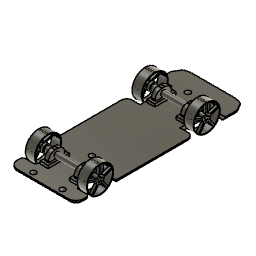
CAR BAse v6 (Autodesk Fusion 360 design; units mm, degrees)
Autodesk Fusion 360 part; units mm, degrees
note: some values were not read from the file. Set by a fixed rule: which face or edge a step refers to.
sketch "Sketch1" plane through (0, 0, 0) normal (0, 0, 1) x (1, 0, 0)
  line L0 (-50, 58.039) -> (-50, 31)
  line L1 (-50, 19) -> (-50, 18)
  line L2 (-47, 15) -> (-28, 15)
  line L3 (-25, 18) -> (-25, 19)
  line L4 (-25, 31) -> (-25, 58)
  line L5 (-25, 70) -> (-25, 70)
  line L6 (-30, 75) -> (-45, 75)
  line L7 (-50, 70) -> (-50, 70)
  arc A0 (-45, 75) -> (-50, 70) centre (-45, 70) ccw
  arc A1 (-25, 70) -> (-30, 75) centre (-30, 70) ccw
  arc A2 (-28, 15) -> (-25, 18) centre (-28, 18) ccw
  arc A3 (-50, 18) -> (-47, 15) centre (-47, 18) ccw
  line L8 (-49, 20) -> (-46, 20)
  line L9 (-45, 21) -> (-45, 29)
  line L10 (-46, 30) -> (-49, 30)
  line L11 (-26, 20) -> (-29, 20)
  line L12 (-30, 21) -> (-30, 30)
  line L13 (-30, 30) -> (-26, 30)
  line L14 (-25, 70) -> (-30, 70)
  line L15 (-30, 70) -> (-30, 60)
  line L16 (-30, 60) -> (-27, 60)
  line L17 (-48, 60.039) -> (-45, 60.039)
  line L18 (-45, 60.039) -> (-45, 70)
  line L19 (-45, 70) -> (-50, 70)
  line L20 (-44, 55) -> (-31, 55)
  line L21 (-31, 55) -> (-31, 35)
  line L22 (-31, 35) -> (-44, 35)
  line L23 (-44, 35) -> (-44, 55)
  circle A4 centre (-43, 28) radius 1
  circle A5 centre (-43, 22) radius 1
  circle A6 centre (-32, 22) radius 1
  circle A7 centre (-32, 28) radius 1
  circle A8 centre (-43, 68) radius 1
  circle A9 centre (-43, 62) radius 1
  circle A10 centre (-32, 62) radius 1
  circle A11 centre (-32, 68) radius 1
  circle A12 centre (-40, 72) radius 1
  circle A13 centre (-35, 72) radius 1
  circle A14 centre (-37.4904, 33.4419) radius 1
  circle A15 centre (-43, 17) radius 1
  circle A16 centre (-32, 17) radius 1
  arc A17 (-48, 60.039) -> (-50, 58.039) centre (-48, 58.039) ccw
  arc A18 (-25, 58) -> (-27, 60) centre (-27, 58) ccw
  arc A19 (-25, 19) -> (-26, 20) centre (-26, 19) ccw
  arc A20 (-26, 30) -> (-25, 31) centre (-26, 31) ccw
  arc A21 (-50, 31) -> (-49, 30) centre (-49, 31) ccw
  arc A22 (-49, 20) -> (-50, 19) centre (-49, 19) ccw
  arc A23 (-46, 20) -> (-45, 21) centre (-46, 21) ccw
  arc A24 (-45, 29) -> (-46, 30) centre (-46, 29) ccw
  arc A25 (-30, 21) -> (-29, 20) centre (-29, 21) ccw
  dimension "d1" = 5
  dimension "d2" = 5
  dimension "d3" = 3
  dimension "d4" = 3
  dimension "d5" = 2
  dimension "d6" = 2
  dimension "d7" = 2
  dimension "d8" = 1
  dimension "d9" = 1
  constraint vertical L0
  constraint parallel L0 L1
  constraint perpendicular L1 L2
  constraint perpendicular L2 L3
  constraint perpendicular L2 L4
  constraint tangent L6 A0
  constraint tangent L6 A1
  constraint tangent L2 A2
  constraint tangent L3 A2
  constraint tangent L1 A3
  constraint tangent L2 A3
  constraint horizontal L8
  constraint vertical L9
  constraint horizontal L10
  constraint horizontal L11
  constraint vertical L12
  constraint horizontal L13
  constraint horizontal L14
  constraint vertical L15
  constraint horizontal L16
  constraint horizontal L17
  constraint vertical L18
  constraint horizontal L19
  constraint coincident A0.centre L18.end
  constraint horizontal L20
  constraint vertical L21
  constraint horizontal L22
  constraint vertical L23
  constraint tangent L17 A17
  constraint tangent L0 A17
  constraint tangent L16 A18
  constraint tangent L4 A18
  constraint tangent L3 A19
  constraint tangent L11 A19
  constraint tangent L13 A20
  constraint tangent L4 A20
  constraint tangent L10 A21
  constraint tangent L0 A21
  constraint equal A20 A21
  constraint tangent L1 A22
  constraint tangent L8 A22
  constraint equal A20 A22
  constraint tangent L8 A23
  constraint tangent L9 A23
  constraint equal A20 A23
  constraint tangent L9 A24
  constraint tangent L10 A24
  constraint equal A20 A24
  constraint tangent L11 A25
  constraint tangent L12 A25
  constraint equal A20 A25
  measures "d1" radius of A0
  measures "d2" radius of A1
  measures "d3" radius of A2
  measures "d4" radius of A3
  measures "d5" diameter of A14
  measures "d6" radius of A17
  measures "d7" radius of A18
  measures "d8" radius of A19
  measures "d9" radius of A20
extrude "Extrude1" add sketch "Sketch1" along normal blind 1.5 makes body 1
sketch "Sketch2" plane through (0, 0, 0) normal (0, 0, 1) x (1, 0, 0)
  circle A0 centre (0, 0) radius 1
  line L0 (0, 0) -> (0, 5)
  circle A1 centre (0, 5) radius 1
  dimension "d12" = 2
  dimension "d13" = 5
  dimension "d14" = 2
  constraint coincident A0.centre L0.start
  constraint vertical L0
  constraint coincident L0.end A1.centre
  measures "d12" diameter of A0
  measures "d13" distance of A0.centre L0.end
  measures "d14" diameter of A1
extrude "Extrude2" add sketch "Sketch2" along normal blind 1.5 separate body makes body 2 at (0.995, 5.0996, 1) makes body 3 at (0.995, -0.0996, 0.5)
sketch "Sketch3" plane through (0, 0, 1.5) normal (0, 0, 1) x (-1, 0, 0)
  circle A0 centre (0, 0) radius 1
  line L0 (-1.5, -6.5) -> (1.5, -6.5)
  line L1 (1.5, -6.5) -> (1.5, 1.5)
  line L2 (1.5, 1.5) -> (-1.5, 1.5)
  line L3 (-1.5, 1.5) -> (-1.5, -6.5)
  dimension "d20" = 3
  dimension "d21" = 8
  constraint perpendicular L0 L1
  constraint perpendicular L1 L2
  constraint perpendicular L0 L3
  measures "d20" distance of L0.start L0.end
  measures "d21" distance of L0.end L1.end
extrude "Extrude3" add sketch "Sketch3" along normal blind 1 contours A0 | L0 L1 L2 L3 bodies 2 3
sketch "Sketch4" plane through (0, 0, 2.5) normal (0, 0, 1) x (-1, 0, 0)
  line L0 (-1.5, 1.5) -> (-1.5, -6.5)
  line L1 (-1.5, -6.5) -> (1.5, -6.5)
  line L2 (1.5, -6.5) -> (1.5, 1.5)
  line L3 (1.5, 1.5) -> (-1.5, 1.5)
  line L4 (0.75, -4.5) -> (0.75, -0.5)
  line L5 (-0.75, -0.5) -> (-0.75, -4.5)
  line L6 (-0.75, -4.5) -> (-0.75, -5.5)
  line L7 (-0.75, -5.5) -> (0.75, -5.5)
  line L8 (0.75, -5.5) -> (0.75, -4.5)
  line L9 (0.75, -0.5) -> (0.75, 0.5)
  line L10 (0.75, 0.5) -> (0, 0.5)
  line L11 (-0.75, -0.5) -> (-0.75, 0.5)
  line L12 (-0.75, 0.5) -> (0, 0.5)
  dimension "d24" = 1
  dimension "d25" = 1.5
  dimension "d26" = 1
  constraint perpendicular L6 L7
  measures "d24" distance of L5.end L6.end
  measures "d25" distance of L6.end L7.end
  measures "d26" distance of L4.end L9.end
extrude "Extrude4" add sketch "Sketch4" along normal blind 3 contours L4 L5 L6 L7 L8 L9 L10 L11 L12 bodies 2
fillet "Fillet1" radius 2.5 2 edges at (0, 5.5, 5.5) (0, -0.5, 5.5) on bodies 2
hole "Hole1" at (-0.75, 2.502, 3.6803) direction (1, 0, 0) diameter 2 depth 2 tip angle 118 bodies 2
copy_body "Body->Comp1" bodies 2 removing the originals makes body 4 in component "tengely tartó"
move_face "MoveFace1" to x (1, 0, 0) y (0, 1, 0) z (0, 0, 1) at (0, 0.5, 0) 1 faces at (0.995, 5.0996, 1) on bodies 4 in component "tengely tartó"
move_face "MoveFace2" to x (1, 0, 0) y (0, 1, 0) z (0, 0, 1) at (0, -0.5, 0) 1 faces at (0.995, -0.0996, 0.5) on bodies 4 in component "tengely tartó"
copy_body "Body->Comp2" bodies 1 removing the originals makes body 5 in component "alap"
move_body "Move1" bodies 5 to x (1, 0, 0) y (0, 1, 0) z (0, 0, 1) at (0, 0, 4) in component "alap"
move_body "Move1'" bodies 4 to x (1, 0, 0) y (0, 1, 0) z (0, 0, 1) at (-21, 25.94, 0) in component "tengely tartó"
move_face "OffsetFaces1" offset 20 1 faces at (-39.6667, 55, 4.5) on bodies 5 in component "alap"
cylinder "CylinderPrimitive1" add diameter 2 height -17 placed x (0, 0, -1) y (0, 1, 0) z (1, 0, 0) at (0, -76.2033, 52.8252) separate body makes body 6
move_face "MoveFace1'" to x (1, 0, 0) y (0, 1, 0) z (0, 0, 1) at (-2, 0, 0) 1 faces at (-11.3333, -76.0051, 53.8054) on bodies 6
move_body "Move1''" bodies 6 to x (1, 0, 0) y (0, 1, 0) z (0, 0, 1) at (-29, 101, -49)
move_body "Move2" bodies 6 to x (1, 0, 0) y (0, 1, 0) z (0, 0, 1) at (0, 0, 8)
copy_body "Body->Comp3" bodies 6 removing the originals makes body 7 in component "tengely"
move_face "MoveFace1''" to x (1, 0, 0) y (0, 1, 0) z (0, 0, 1) at (0, 0, -8) 1 faces at (-34.6667, 24.6972, 10.8302) on bodies 7 in component "tengely"
sketch "Sketch6" plane through (-29, 0, 0) normal (1, 0, 0) x (0, 1, 0)
  circle A0 centre (65.0267, 3.6652) radius 1
sketch "Sketch7" plane through (0, 0, 0) normal (0, 0, 1) x (1, 0, 0)
  circle A0 centre (0, 0) radius 5
  line L0 (0, 0) -> (5, 0) construction
  line L1 (0, 0) -> (-5, 0) construction
  line L2 (-2.4394, 0.5823) -> (-4.5237, 1.4488)
  line L3 (-4.5113, 1.4868) -> (-2.3158, 0.9628)
  line L4 (-2.4394, 0.5823) -> (-1.459, 0.3483)
  line L5 (-1.3851, 0.5758) -> (-2.3158, 0.9628)
  line L6 (-1.6313, -1.905) -> (-2.8081, -3.831)
  line L7 (-2.7758, -3.8546) -> (-1.3077, -2.1401)
  line L8 (-1.3077, -2.1401) -> (-0.7821, -1.28)
  line L9 (-0.9756, -1.1394) -> (-1.6313, -1.905)
  line L10 (1.3077, -2.1401) -> (2.7758, -3.8546)
  line L11 (2.8081, -3.831) -> (1.6313, -1.905)
  line L12 (1.3077, -2.1401) -> (0.7821, -1.28)
  line L13 (0.9756, -1.1394) -> (1.6313, -1.905)
  line L14 (-0.2, 2.5) -> (-0.1196, 1.4952)
  line L15 (0.1196, 1.4952) -> (0.2, 2.5)
  line L16 (0.2, 2.5) -> (0.02, 4.75)
  line L17 (-0.02, 4.75) -> (-0.2, 2.5)
  line L18 (2.3158, 0.9628) -> (1.3851, 0.5758)
  line L19 (1.459, 0.3483) -> (2.4394, 0.5823)
  line L20 (2.4394, 0.5823) -> (4.5237, 1.4488)
  line L21 (4.5113, 1.4868) -> (2.3158, 0.9628)
  line L22 (0.5701, 0.1853) -> (0, 0)
  circle A1 centre (-0.7133, -0.2318) radius 0.25
  circle A2 centre (0, -0.75) radius 0.25
  circle A3 centre (0.7133, -0.2318) radius 0.25
  circle A4 centre (0.4566, 0.595) radius 0.25
  circle A5 centre (-0.4408, 0.6068) radius 0.25
  arc A6 (-0.7821, -1.28) -> (0.7821, -1.28) centre (0, 0) ccw
  arc A7 (0.9756, -1.1394) -> (1.459, 0.3483) centre (0, 0) ccw
  arc A8 (1.3851, 0.5758) -> (0.1196, 1.4952) centre (0, 0) ccw
  arc A9 (-0.1196, 1.4952) -> (-1.3851, 0.5758) centre (0, 0) ccw
  arc A10 (-1.459, 0.3483) -> (-0.9756, -1.1394) centre (0, 0) ccw
  arc A11 (-0.02, 4.75) -> (-4.5113, 1.4868) centre (0, 0) ccw
  arc A12 (4.5113, 1.4868) -> (0.02, 4.75) centre (0, 0) ccw
  arc A13 (2.8081, -3.831) -> (4.5237, 1.4488) centre (0, 0) ccw
  arc A14 (-4.5237, 1.4488) -> (-2.8081, -3.831) centre (0, 0) ccw
  arc A15 (-2.7758, -3.8546) -> (2.7758, -3.8546) centre (0, 0) ccw
  dimension "d50" = 10
  dimension "d54" = 3
  dimension "d61" = 9.5
  dimension "d73" = 0.75
  dimension "d74" = 0.5
  dimension "d75" = 0.5
  dimension "d76" = 0.5
  dimension "d77" = 0.5
  dimension "d78" = 0.5
  constraint coincident A0.centre L0.start
  constraint concentric A0 A6
  constraint horizontal L0
  constraint horizontal L1
  constraint concentric A6 A14
  constraint coincident L17.start A14
  constraint coincident L21.start A14
  constraint coincident L11.start A14
  constraint coincident L7.start A14
  constraint coincident L4.end A6
  constraint coincident L5.start A6
  constraint coincident L15.start A6
  constraint coincident L14.end A6
  constraint coincident L18.end A6
  constraint coincident L19.start A6
  constraint coincident L13.start A6
  constraint concentric A6 A7
  constraint concentric A7 A8
  constraint concentric A8 A9
  constraint concentric A9 A10
  constraint concentric A11 A14
  constraint concentric A12 A14
  constraint concentric A13 A14
  constraint concentric A14 A15
  measures "d50" diameter of A0
  measures "d54" diameter of A6
  measures "d61" diameter of A14
  measures "d73" distance of A0.centre A1.centre
  measures "d74" diameter of A1
  measures "d75" diameter of A2
  measures "d76" diameter of A3
  measures "d77" diameter of A4
  measures "d78" diameter of A5
sketch "Sketch8" plane through (0, 0, 0.5) normal (0, 0, 1) x (-1, 0, 0)
  circle A0 centre (0.7133, 0.2318) radius 0.25
  line L0 (2.7758, 3.8546) -> (1.3077, 2.1401)
  line L1 (1.3077, 2.1401) -> (0.7821, 1.28)
  arc A1 (0.7821, 1.28) -> (-0.7821, 1.28) centre (0, 0) ccw
  line L2 (-0.7821, 1.28) -> (-1.3077, 2.1401)
  line L3 (-1.3077, 2.1401) -> (-2.7758, 3.8546)
  arc A2 (2.7758, 3.8546) -> (-2.7758, 3.8546) centre (0, 0) ccw
  line L4 (4.5237, -1.4488) -> (2.4394, -0.5823)
  line L5 (2.4394, -0.5823) -> (1.459, -0.3483)
  arc A3 (1.459, -0.3483) -> (0.9756, 1.1394) centre (0, 0) ccw
  line L6 (0.9756, 1.1394) -> (1.6313, 1.905)
  line L7 (1.6313, 1.905) -> (2.8081, 3.831)
  arc A4 (4.5237, -1.4488) -> (2.8081, 3.831) centre (0, 0) ccw
  line L8 (-1.6313, 1.905) -> (-0.9756, 1.1394)
  arc A5 (-0.9756, 1.1394) -> (-1.459, -0.3483) centre (0, 0) ccw
  line L9 (-1.459, -0.3483) -> (-2.4394, -0.5823)
  line L10 (-2.4394, -0.5823) -> (-4.5237, -1.4488)
  arc A6 (-2.8081, 3.831) -> (-4.5237, -1.4488) centre (0, 0) ccw
  line L11 (-2.8081, 3.831) -> (-1.6313, 1.905)
  line L12 (-4.5113, -1.4868) -> (-2.3158, -0.9628)
  line L13 (-2.3158, -0.9628) -> (-1.3851, -0.5758)
  arc A7 (-1.3851, -0.5758) -> (-0.1196, -1.4952) centre (0, 0) ccw
  line L14 (-0.1196, -1.4952) -> (-0.2, -2.5)
  line L15 (-0.2, -2.5) -> (-0.02, -4.75)
  arc A8 (-4.5113, -1.4868) -> (-0.02, -4.75) centre (0, 0) ccw
  line L16 (0.02, -4.75) -> (0.2, -2.5)
  line L17 (0.2, -2.5) -> (0.1196, -1.4952)
  arc A9 (0.1196, -1.4952) -> (1.3851, -0.5758) centre (0, 0) ccw
  line L18 (1.3851, -0.5758) -> (2.3158, -0.9628)
  line L19 (2.3158, -0.9628) -> (4.5113, -1.4868)
  arc A10 (0.02, -4.75) -> (4.5113, -1.4868) centre (0, 0) ccw
  circle A11 centre (0.4408, -0.6068) radius 0.25
  circle A12 centre (-0.4566, -0.595) radius 0.25
  circle A13 centre (-0.7133, 0.2318) radius 0.25
  circle A14 centre (0, 0.75) radius 0.25
  circle A15 centre (0, 0) radius 5
  line L20 (2.8081, 3.831) -> (2.7758, 3.8546)
  line L21 (-2.7758, 3.8546) -> (-2.8081, 3.831)
  line L22 (-4.5113, -1.4868) -> (-4.5237, -1.4488)
  line L23 (0.02, -4.75) -> (-0.02, -4.75)
  line L24 (4.5113, -1.4868) -> (4.5237, -1.4488)
  line L25 (1.459, -0.3483) -> (1.3851, -0.5758)
  line L26 (0.1196, -1.4952) -> (-0.1196, -1.4952)
  line L27 (-1.3851, -0.5758) -> (-1.459, -0.3483)
  line L28 (-0.9756, 1.1394) -> (-0.7821, 1.28)
  line L29 (0.7821, 1.28) -> (0.9756, 1.1394)
  constraint coincident L7.end A4.end
  constraint coincident L0.start A2.start
  constraint coincident L3.end A2.end
  constraint coincident A6.start L11.start
  constraint coincident L12.start A8.start
  constraint coincident L10.end A6.end
  constraint coincident L16.start A10.start
  constraint coincident L15.end A8.end
  constraint horizontal L23
  constraint coincident L19.end A10.end
  constraint coincident L4.start A4.start
  constraint coincident L5.end A3.start
  constraint coincident A9.end L18.start
  constraint coincident L17.end A9.start
  constraint coincident A7.end L14.start
  constraint coincident L13.end A7.start
  constraint coincident A5.end L9.start
  constraint coincident L8.end A5.start
  constraint coincident A1.end L2.start
  constraint coincident L1.end A1.start
  constraint coincident A3.end L6.start
sketch "Sketch9" plane through (0, 0, 1.8) normal (0, 0, 1) x (-1, 0, 0)
  arc A0 (0.02, -4.75) -> (4.5113, -1.4868) centre (0, 0) ccw
  line L0 (0.02, -4.75) -> (-0.02, -4.75)
  arc A1 (-4.5113, -1.4868) -> (-0.02, -4.75) centre (0, 0) ccw
  line L1 (-4.5113, -1.4868) -> (-4.5237, -1.4488)
  arc A2 (-2.8081, 3.831) -> (-4.5237, -1.4488) centre (0, 0) ccw
  line L2 (-2.8081, 3.831) -> (-2.7758, 3.8546)
  arc A3 (2.7758, 3.8546) -> (-2.7758, 3.8546) centre (0, 0) ccw
  line L3 (2.7758, 3.8546) -> (2.8081, 3.831)
  arc A4 (4.5237, -1.4488) -> (2.8081, 3.831) centre (0, 0) ccw
  line L4 (4.5237, -1.4488) -> (4.5113, -1.4868)
  circle A5 centre (0, 0) radius 5
sketch "Sketch10" plane through (-29, 0, 0) normal (1, 0, 0) x (0, 1, 0)
  circle A0 centre (25.0267, 3.6652) radius 1
  circle A1 centre (25.0267, 3.6652) radius 1.5
  line L0 (26.0267, 3.6652) -> (26.5267, 3.6652) construction
  dimension "d85" = 3
  constraint concentric A0 A1
  constraint horizontal L0
  constraint coincident A0 L0.start
  measures "d85" diameter of A1
extrude "Extrude1'" add sketch "Sketch10" along normal blind 1 contours A0 | A1 sketch seen with x (1, 0, 0) y (0, 1, 0) z (0, 0, 1) at (0, -0.23, 0.16) bodies 7 in component "tengely"
sketch "Sketch11" plane through (-28, 0, 0) normal (1, 0, 0) x (0, 1, 0)
  circle A0 centre (25.0267, 3.6652) radius 1.5
sketch "Sketch12" plane through (-46, 0, 0) normal (-1, 0, 0) x (0, -1, 0)
  circle A0 centre (-25.0267, 3.6652) radius 1
  circle A1 centre (-25.0267, 3.6652) radius 1.5
  dimension "d95" = 3
  constraint concentric A0 A1
  measures "d95" diameter of A1
extrude "Extrude2'" add sketch "Sketch12" along normal blind 1 contours A0 | A1 sketch seen with x (1, 0, 0) y (0, 1, 0) z (0, 0, 1) at (0, -0.23, 0.16) bodies 7 in component "tengely"
sketch "Sketch13" plane through (-28, 0, 0) normal (1, 0, 0) x (0, 1, 0)
  circle A0 centre (65.0267, 3.6652) radius 1.5
  line L0 (65.0267, 3.6652) -> (66.5267, 3.6652) construction
  line L1 (65.0267, 3.6652) -> (66.5267, 3.6652) construction
  line L2 (65.0267, 3.6652) -> (66.5267, 3.6652) construction
  line L3 (65.0267, 3.6652) -> (65.0267, 4.4152)
  line L4 (65.0267, 3.6652) -> (65.74, 3.897)
  line L5 (65.0267, 3.6652) -> (65.4673, 3.0583)
  line L6 (65.0267, 3.6652) -> (64.5862, 3.0583)
  line L7 (65.0267, 3.6652) -> (64.3135, 3.8974)
  circle A1 centre (64.5862, 3.0583) radius 0.25
  circle A2 centre (65.4673, 3.0583) radius 0.25
  circle A3 centre (65.0267, 4.4152) radius 0.25
  circle A4 centre (65.74, 3.897) radius 0.25
  circle A5 centre (64.3135, 3.8974) radius 0.25
  dimension "d107" = 0.5
  dimension "d108" = 0.5
  dimension "d110" = 0.5
  dimension "d111" = 0.5
  dimension "d112" = 0.5
  constraint coincident A0.centre L0.start
  constraint horizontal L0
  constraint horizontal L1
  constraint horizontal L2
  constraint coincident L6.end A1.centre
  constraint coincident L5.end A2.centre
  constraint coincident L3.end A3.centre
  constraint coincident L4.end A4.centre
  constraint coincident L7.end A5.centre
  measures "d107" diameter of A1
  measures "d108" diameter of A2
  measures "d110" diameter of A3
  measures "d111" diameter of A4
  measures "d112" diameter of A5
extrude "Extrude3'" add sketch "Sketch13" along normal blind 1.5 contours A1 | A2 | A3 | A4 | A5 sketch seen with x (1, 0, 0) y (0, 1, 0) z (0, 0, 1) at (0, -40.23, 0.16) bodies 7 in component "tengely"
sketch "Sketch14" plane through (-47, 0, 0) normal (-1, 0, 0) x (0, -1, 0)
  circle A0 centre (-65.0267, 3.6652) radius 1.5
  line L0 (-65.0267, 3.6652) -> (-65.0267, 4.4152)
  line L1 (-65.0267, 3.6652) -> (-65.74, 3.8969)
  line L2 (-65.0267, 3.6652) -> (-65.468, 3.0588)
  line L3 (-65.0267, 3.6652) -> (-64.5854, 3.0588)
  line L4 (-65.0267, 3.6652) -> (-64.3134, 3.8969)
  circle A1 centre (-65.468, 3.0588) radius 0.25
  circle A2 centre (-64.5854, 3.0588) radius 0.25
  circle A3 centre (-64.3134, 3.8969) radius 0.25
  circle A4 centre (-65.0267, 4.4152) radius 0.25
  circle A5 centre (-65.74, 3.8969) radius 0.25
  dimension "d116" = 0.5
  dimension "d117" = 0.5
  dimension "d118" = 0.5
  dimension "d119" = 0.5
  dimension "d120" = 0.5
  constraint coincident A0.centre L0.start
  constraint coincident L2.end A1.centre
  constraint coincident L3.end A2.centre
  constraint coincident L4.end A3.centre
  constraint coincident L0.end A4.centre
  constraint coincident L1.end A5.centre
  measures "d116" diameter of A1
  measures "d117" diameter of A2
  measures "d118" diameter of A3
  measures "d119" diameter of A4
  measures "d120" diameter of A5
extrude "Extrude4'" add sketch "Sketch14" along normal blind 1.5 contours A1 | A2 | A3 | A4 | A5 sketch seen with x (1, 0, 0) y (0, 1, 0) z (0, 0, 1) at (0, -40.23, 0.16) bodies 7 in component "tengely"
sketch "Sketch15" plane through (0, 0, 0) normal (0, 0, 1) x (1, 0, 0)
  circle A0 centre (0, 0) radius 5
  circle A1 centre (-0.6075, -0.4398) radius 0.25
  circle A2 centre (0.2311, -0.7135) radius 0.25
  circle A3 centre (-0.6063, 0.4414) radius 0.25
  circle A4 centre (0.2324, 0.7131) radius 0.25
  circle A5 centre (0.75, 0) radius 0.25
  line L0 (-3.6639, -3.0229) -> (-1.0156, -1.1039)
  line L1 (0.737, -1.3065) -> (1.7462, -4.4174)
  line L2 (1.1758, -4.6022) -> (0.1691, -1.4904)
  line L3 (4.7406, 0.2985) -> (1.47, 0.2985)
  line L4 (1.47, -0.2985) -> (4.7406, -0.2985)
  line L5 (1.1836, 4.6002) -> (0.1716, 1.4902)
  line L6 (0.7392, 1.3052) -> (1.7536, 4.4144)
  line L7 (-3.656, 3.0325) -> (-1.0127, 1.1065)
  line L8 (-1.3641, 0.6239) -> (-4.0089, 2.5478)
  line L9 (-4.0156, -2.5372) -> (-1.3657, -0.6203)
  arc A6 (-1.3641, 0.6239) -> (-1.3657, -0.6203) centre (0, 0) ccw
  arc A7 (-4.0089, 2.5478) -> (-4.0156, -2.5372) centre (0, 0) ccw
  arc A8 (0.1716, 1.4902) -> (-1.0127, 1.1065) centre (0, 0) ccw
  arc A9 (1.47, 0.2985) -> (0.7392, 1.3052) centre (0, 0) ccw
  arc A10 (4.7406, 0.2985) -> (1.7536, 4.4144) centre (0, 0) ccw
  arc A11 (1.1836, 4.6002) -> (-3.656, 3.0325) centre (0, 0) ccw
  arc A12 (-3.6639, -3.0229) -> (1.1758, -4.6022) centre (0, 0) ccw
  arc A13 (1.7462, -4.4174) -> (4.7406, -0.2985) centre (0, 0) ccw
  arc A14 (-1.0156, -1.1039) -> (0.1691, -1.4904) centre (0, 0) ccw
  arc A15 (0.737, -1.3065) -> (1.47, -0.2985) centre (0, 0) ccw
  dimension "d123" = 3
  dimension "d124" = 10
  dimension "d125" = 9.5
  dimension "d126" = 0.5
  dimension "d127" = 0.75
  dimension "d128" = 0.75
  dimension "d129" = 0.75
  dimension "d130" = 0.75
  dimension "d131" = 0.5
  dimension "d132" = 0.5
  dimension "d133" = 0.5
  dimension "d134" = 0.5
  constraint coincident A0.centre A6.centre
  constraint concentric A0 A14
  constraint concentric A0 A12
  constraint coincident L1.start A14
  constraint coincident L3.end A14
  constraint parallel L3 L4
  constraint coincident L5.end A14
  constraint coincident L8.start A14
  constraint concentric A6 A14
  constraint concentric A7 A12
  constraint concentric A8 A14
  constraint concentric A9 A14
  constraint concentric A10 A12
  constraint concentric A10 A11
  constraint concentric A12 A13
  constraint concentric A14 A15
  measures "d123" diameter of A14
  measures "d124" diameter of A0
  measures "d125" diameter of A12
  measures "d126" diameter of A1
  measures "d127" distance of A0.centre A2.centre
  measures "d128" distance of A0.centre A5.centre
  measures "d129" distance of A0.centre A4.centre
  measures "d130" distance of A0.centre A3.centre
  measures "d131" diameter of A2
  measures "d132" diameter of A3
  measures "d133" diameter of A4
  measures "d134" diameter of A5
extrude "Extrude8" add sketch "Sketch15" along normal blind 1 separate body makes body 8
sketch "Sketch16" plane through (0, 0, 1) normal (0, 0, 1) x (-1, 0, 0)
  arc A0 (-1.7462, 4.4174) -> (-4.7406, 0.2985) centre (0, 0) ccw
  line L0 (-1.7462, 4.4174) -> (-0.737, 1.3065)
  arc A1 (-0.737, 1.3065) -> (-1.47, 0.2985) centre (0, 0) ccw
  line L1 (-1.47, 0.2985) -> (-4.7406, 0.2985)
  arc A2 (3.6639, 3.0229) -> (-1.1758, 4.6022) centre (0, 0) ccw
  line L2 (3.6639, 3.0229) -> (1.0156, 1.1039)
  arc A3 (1.0156, 1.1039) -> (-0.1691, 1.4904) centre (0, 0) ccw
  line L3 (-0.1691, 1.4904) -> (-1.1758, 4.6022)
  line L4 (-1.1836, -4.6002) -> (-0.1716, -1.4902)
  arc A4 (-0.1716, -1.4902) -> (1.0127, -1.1065) centre (0, 0) ccw
  line L5 (1.0127, -1.1065) -> (3.656, -3.0325)
  arc A5 (-1.1836, -4.6002) -> (3.656, -3.0325) centre (0, 0) ccw
  line L6 (-4.7406, -0.2985) -> (-1.47, -0.2985)
  arc A6 (-1.47, -0.2985) -> (-0.7392, -1.3052) centre (0, 0) ccw
  line L7 (-0.7392, -1.3052) -> (-1.7536, -4.4144)
  arc A7 (-4.7406, -0.2985) -> (-1.7536, -4.4144) centre (0, 0) ccw
  line L8 (4.0089, -2.5478) -> (1.3641, -0.6239)
  arc A8 (1.3641, -0.6239) -> (1.3657, 0.6203) centre (0, 0) ccw
  line L9 (1.3657, 0.6203) -> (4.0156, 2.5372)
  arc A9 (4.0089, -2.5478) -> (4.0156, 2.5372) centre (0, 0) ccw
  circle A10 centre (-0.75, 0) radius 0.25
  circle A11 centre (-0.2324, -0.7131) radius 0.25
  circle A12 centre (0.6063, -0.4414) radius 0.25
  circle A13 centre (-0.2311, 0.7135) radius 0.25
  circle A14 centre (0.6075, 0.4398) radius 0.25
  circle A15 centre (0, 0) radius 5
  line L10 (4.0156, 2.5372) -> (3.6639, 3.0229)
  line L11 (-1.1758, 4.6022) -> (-1.7462, 4.4174)
  line L12 (-4.7406, 0.2985) -> (-4.7406, -0.2985)
  line L13 (-1.7536, -4.4144) -> (-1.1836, -4.6002)
  line L14 (3.656, -3.0325) -> (4.0089, -2.5478)
  line L15 (1.3641, -0.6239) -> (1.0127, -1.1065)
  line L16 (-0.1716, -1.4902) -> (-0.7392, -1.3052)
  line L17 (-1.47, -0.2985) -> (-1.47, 0.2985)
  line L18 (-0.737, 1.3065) -> (-0.1691, 1.4904)
  line L19 (1.0156, 1.1039) -> (1.3657, 0.6203)
  constraint coincident L9.end A9.end
  constraint coincident A2.start L2.start
  constraint coincident A2.end L3.end
  constraint coincident A0.start L0.start
  constraint coincident A0.end L1.end
  constraint coincident L6.start A7.start
  constraint coincident L7.end A7.end
  constraint coincident L4.start A5.start
  constraint coincident L5.end A5.end
  constraint coincident L8.start A9.start
  constraint coincident L8.end A8.start
  constraint coincident A4.end L5.start
  constraint coincident L4.end A4.start
  constraint coincident A6.end L7.start
  constraint coincident L6.end A6.start
  constraint coincident A1.end L1.start
  constraint coincident L0.end A1.start
  constraint coincident A3.end L3.start
  constraint coincident L2.end A3.start
  constraint coincident A8.end L9.start
extrude "Extrude9" add sketch "Sketch16" along normal blind 1 contours A1 A3 A4 A6 A8 L15 L16 L17 L18 L19 | A15 bodies 8
sketch "Sketch17" plane through (0, 0, 2) normal (0, 0, 1) x (-1, 0, 0)
  line L0 (4.0089, -2.5478) -> (3.656, -3.0325)
  arc A0 (-1.1836, -4.6002) -> (3.656, -3.0325) centre (0, 0) ccw
  line L1 (-1.1836, -4.6002) -> (-1.7536, -4.4144)
  arc A1 (-4.7406, -0.2985) -> (-1.7536, -4.4144) centre (0, 0) ccw
  line L2 (-4.7406, -0.2985) -> (-4.7406, 0.2985)
  arc A2 (-1.7462, 4.4174) -> (-4.7406, 0.2985) centre (0, 0) ccw
  line L3 (-1.7462, 4.4174) -> (-1.1758, 4.6022)
  arc A3 (3.6639, 3.0229) -> (-1.1758, 4.6022) centre (0, 0) ccw
  line L4 (3.6639, 3.0229) -> (4.0156, 2.5372)
  arc A4 (4.0089, -2.5478) -> (4.0156, 2.5372) centre (0, 0) ccw
  circle A5 centre (0, 0) radius 5
extrude "Extrude10" add sketch "Sketch17" along normal blind 2.5 bodies 8
copy_body "Body->Comp5" bodies 8 removing the originals makes body 9 in component "kerék"
move_face "OffsetFaces2" offset -1 1 faces at (-29, 60, 4.5) on bodies 5 in component "alap"
move_face "OffsetFaces3" offset 4 1 faces at (-35, 75, 5) on bodies 5 in component "alap"
move_face "OffsetFaces4" offset -1 2 faces at (-48, 70, 4.5) (-24, 70, 4.5) on bodies 5 in component "alap"
sketch "Sketch18" plane through (0, 0, 1.5) normal (0, 0, 1) x (-1, 0, 0)
  circle A0 centre (32, -22) radius 1
  circle A1 centre (43, -22) radius 1
  circle A2 centre (43, -28) radius 1
  circle A3 centre (32, -28) radius 1
  circle A4 centre (43, -68) radius 1
  circle A5 centre (43, -62) radius 1
  circle A6 centre (32, -62) radius 1
  circle A7 centre (32, -68) radius 1
  circle A8 centre (40, -72) radius 1
  circle A9 centre (35, -72) radius 1
  circle A10 centre (37.4904, -33.4419) radius 1
  circle A11 centre (43, -17) radius 1
  circle A12 centre (32, -17) radius 1
  arc A13 (25, -57) -> (27, -59) centre (27, -57) ccw
  line L0 (27, -59) -> (30, -59)
  line L1 (30, -59) -> (30, -71)
  line L2 (30, -71) -> (21.0557, -71)
  arc A14 (21.0557, -71) -> (30, -79) centre (30, -70) ccw
  line L3 (30, -79) -> (45, -79)
  arc A15 (45, -79) -> (53.9443, -71) centre (45, -70) ccw
  line L4 (53.9443, -71) -> (45, -71)
  line L5 (45, -71) -> (45, -60.039)
  line L6 (45, -60.039) -> (48, -60.039)
  arc A16 (48, -60.039) -> (50, -58.039) centre (48, -58.039) ccw
  line L7 (50, -58.039) -> (50, -31)
  arc A17 (50, -31) -> (49, -30) centre (49, -31) ccw
  line L8 (49, -30) -> (46, -30)
  arc A18 (45, -29) -> (46, -30) centre (46, -29) ccw
  line L9 (45, -29) -> (45, -21)
  arc A19 (46, -20) -> (45, -21) centre (46, -21) ccw
  line L10 (46, -20) -> (49, -20)
  arc A20 (49, -20) -> (50, -19) centre (49, -19) ccw
  line L11 (50, -19) -> (50, -18)
  arc A21 (50, -18) -> (47, -15) centre (47, -18) ccw
  line L12 (47, -15) -> (28, -15)
  arc A22 (28, -15) -> (25, -18) centre (28, -18) ccw
  line L13 (25, -18) -> (25, -19)
  arc A23 (25, -19) -> (26, -20) centre (26, -19) ccw
  line L14 (26, -20) -> (29, -20)
  arc A24 (30, -21) -> (29, -20) centre (29, -21) ccw
  line L15 (30, -21) -> (30, -30)
  line L16 (30, -30) -> (26, -30)
  arc A25 (26, -30) -> (25, -31) centre (26, -31) ccw
  line L17 (25, -31) -> (25, -57)
  line L18 (50, -71) -> (50, -78.4784)
  line L19 (50, -78.4784) -> (45.9302, -80.226)
  line L20 (45.9302, -80.226) -> (33.6049, -81.2837)
  line L21 (33.6049, -81.2837) -> (25, -77.9725)
  line L22 (25, -71) -> (25, -77.9725)
  line L23 (25, -71) -> (23.7631, -68.4526)
  line L24 (23.7631, -68.4526) -> (14.4272, -70.4762)
  line L25 (14.4272, -70.4762) -> (19.532, -79.8581)
  line L26 (19.532, -79.8581) -> (32.2252, -82.4795)
  line L27 (32.2252, -82.4795) -> (43.9998, -84.9112)
  line L28 (43.9998, -84.9112) -> (50.8511, -83.6953)
  line L29 (50.8511, -83.6953) -> (54.8062, -79.8581)
  line L30 (54.8062, -79.8581) -> (54.8062, -74.3853)
  line L31 (54.8062, -74.3853) -> (54.8062, -69.9703)
  line L32 (54.8062, -69.9703) -> (50.2992, -67.8547)
  line L33 (50.2992, -67.8547) -> (50, -71)
  constraint parallel L7 L18
  constraint coincident L2 L22.start
  constraint coincident L4 L18.start
  constraint parallel L26 L27
  constraint vertical L30
  constraint parallel L30 L31
extrude "Extrude1''" cut sketch "Sketch18" against normal blind 3 contours L2 A14 L22 | L2 A14 A15 L4 L18 L19 L20 L21 L22 L23 L24 L25 L26 L27 L28 L29 L30 L31 L32 L33 | A15 L4 L18 sketch seen with x (1, 0, 0) y (0, 1, 0) z (0, 0, 1) at (0, 0, 4) bodies 5 in component "alap"
chamfer "Chamfer1" distance 2 angle 45 2 edges at (-25, 77.4833, 4.75) (-50, 77.4833, 4.75) on bodies 5 in component "alap"
chamfer "Chamfer2" distance 1 angle 45 7 edges at (-25.8881, 76.943, 4) (-28.3606, 78.8494, 4) (-37.5, 79, 4) (-46.6394, 78.8494, 4) (-49.1119, 76.943, 4) (-50, 73.2417, 4) (-25, 73.2417, 4) on bodies 5 in component "alap"
move_face "OffsetFaces1'" offset -1 1 faces at (-2.417, 4.1765, 4.5) on bodies 9 in component "kerék"
move_face "OffsetFaces5" offset -1 1 faces at (-46, 60.039, 5) on bodies 5 in component "alap"
chamfer "Chamfer3" distance 1 angle 45 19 edges at (-50, 44.0195, 4) (-49.7071, 30.2929, 4) (-47.5, 30, 4) (-45.2929, 29.7071, 4) (-45, 25, 4) (-45.2929, 20.2929, 4) (-47.5, 20, 4) (-49.7071, 19.7071, 4) (-50, 18.5, 4) (-49.1213, 15.8787, 4) (-37.5, 15, 4) (-25.8787, 15.8787, 4) (-25, 18.5, 4) (-25.2929, 19.7071, 4) (-27.5, 20, 4) (-29.7071, 20.2929, 4) (-30, 25.5, 4) (-46.5, 59.039, 4) (-49.4142, 58.4532, 4) on bodies 5 in component "alap"
chamfer "Chamfer4" distance 1 angle 45 5 edges at (-25, 44, 4) (-25.5858, 58.4142, 4) (-28.5, 59, 4) (-28.5, 30, 4) (-25.2929, 30.2929, 4) on bodies 5 in component "alap"
component "alap" placed x (1, 0, 0) y (0, 1, 0) z (0, 0, 1) at (0, 0, -4)
component "tengely tartó" placed x (1, 0, 0) y (0, 1, 0) z (0, 0, 1) at (-10.996, -3.4128, -0.0134)
component "tengely tartó" placed x (1, 0, 0) y (0, 1, 0) z (0, 0, 1) at (-21.996, -3.4128, -0.0134)
component "tengely tartó" placed x (1, 0, 0) y (0, 1, 0) z (0, 0, 1) at (-10.996, 36.5872, -0.0134)
component "tengely tartó" placed x (1, 0, 0) y (0, 1, 0) z (0, 0, 1) at (-21.996, 36.5872, -0.0134)
component "tengely" placed x (1, 0, 0) y (0, 1, 0) z (0, 0, 1) at (0, 0.23, -0.16)
component "tengely" placed x (1, 0, 0) y (0, 1, 0) z (0, 0, 1) at (0, 40.23, -0.16)
component "kerék" placed x (0, 0, 1) y (0, 1, 0) z (-1, 0, 0) at (-26.0127, 25.03, 3.6874)
component "kerék" placed x (0, 0, 1) y (0, 1, 0) z (-1, 0, 0) at (-26.0127, 65.03, 3.6874)
component "kerék" placed x (0, 0, 1) y (0, -1, 0) z (1, 0, 0) at (-48.9874, 65.0303, 3.6874)
component "kerék" placed x (0, 0, 1) y (0, -1, 0) z (1, 0, 0) at (-48.9874, 25.0303, 3.6874)
